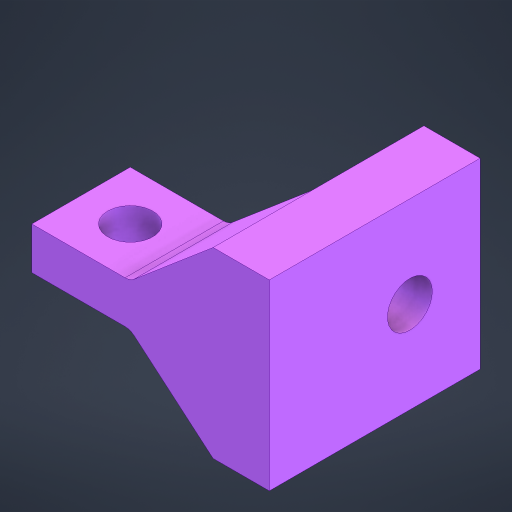
# Autodesk Inventor part: base_servos
Saved by Autodesk Inventor 2023.1 (Build 271208000, 208)
## iProperties
Created: 2022-11-08
Part Number: base_servos
Material: Generic
Document SubType Name: Modeling
Designer: amtat
Density: 1 g/cm^3
Appearance: Default
Author: amtat
Autodesk Inventor part; units mm, degrees
ref_plane "YZ Plane" through (0, 0, 0) normal (1, 0, 0) x (0, 1, 0)
ref_plane "XZ Plane" through (0, 0, 0) normal (0, 1, 0) x (-1, 0, 0)
ref_plane "XY Plane" through (0, 0, 0) normal (0, 0, 1) x (1, 0, 0)
sketch "Sketch1" plane through (0, 0, 0) normal (1, 0, 0) x (0, 1, 0)
  circle A0 centre (0, 0) radius 1.6
  line L0 (0, 0) -> (0, -66.3)
  circle A1 centre (0, -66.3) radius 1.6
  line L1 (0, 0) -> (3.5, 0)
  line L2 (3.5, 0) -> (3.5, 3.5)
  line L3 (3.5, 3.5) -> (-3.5, 3.5)
  line L4 (-3.5, 3.5) -> (-3.5, -3.5)
  line L5 (-3.5, -3.5) -> (3.5, -3.5)
  line L6 (3.5, -3.5) -> (3.5, 0)
  line L7 (0, -66.3) -> (3.5, -66.3)
  line L8 (3.5, -66.3) -> (3.5, -62.8)
  line L9 (3.5, -62.8) -> (-3.5, -62.8)
  line L10 (-3.5, -62.8) -> (-3.5, -69.8)
  line L11 (-3.5, -69.8) -> (3.5, -69.8)
  line L12 (3.5, -69.8) -> (3.5, -66.3)
  line L13 (3.5, 3.5) -> (3.5, 6.5)
  line L14 (3.5, 6.5) -> (-3.5, 6.5)
  line L15 (-3.5, 6.5) -> (-3.5, 3.5)
  line L16 (3.5, -69.8) -> (3.5, -72.8)
  line L17 (3.5, -72.8) -> (-3.5, -72.8)
  line L18 (-3.5, -72.8) -> (-3.5, -69.8)
  dimension "d0" = 3.2
  dimension "d1" = 66.3
  dimension "d2" = 3.2
  dimension "d3" = 3.5
  dimension "d4" = 3.5
  dimension "d5" = 7
  dimension "d6" = 7
  dimension "d7" = 3.5
  dimension "d8" = 3.5
  dimension "d9" = 7
  dimension "d10" = 7
  dimension "d11" = 3
  dimension "d12" = 3
  constraints: 38 end point, 11 perpendicular, 8 point on line, 2 centre point, 2 coincident, 2 vertical, 1 horizontal
  measures "d0" diameter of A0
  measures "d1" distance of L0.start L0.end
  measures "d2" diameter of A1
  measures "d3" distance of L0.start L1.end
  measures "d4" distance of L1.end L2.end
  measures "d5" distance of L2.end L3.end
  measures "d6" distance of L3.end L4.end
  measures "d7" distance of L7.start L7.end
  measures "d8" distance of L7.end L8.end
  measures "d9" distance of L8.end L9.end
  measures "d10" distance of L9.end L10.end
  measures "d11" distance of L2.end L13.end
  measures "d12" distance of L11.end L16.end
extrude "Extrusion1" add sketch "Sketch1" along normal blind 3 contours L1 L6 L5 L0 A0 | A0 L0 L5 L4 L3 L2 L1 | L3 L15 L14 L13 | L9 L8 L7 A1 L0 | L0 A1 L7 L12 L11 L10 L9 | L11 L16 L17 L18
sketch "Sketch2" plane through (3, 0, 0) normal (1, 0, 0) x (0, 0, -1)
  line L0 (-6.5, 3.5) -> (-6.5, -3.5) projected
  line L1 (-6.5, -3.5) -> (3.5, -3.5) projected
  line L2 (3.5, -3.5) -> (3.5, 3.5) projected
  line L3 (3.5, 3.5) -> (-6.5, 3.5) projected
  circle A0 centre (0, 0) radius 1.6 projected
  line L4 (62.8, -3.5) -> (72.8, -3.5) projected
  line L5 (72.8, -3.5) -> (72.8, 3.5) projected
  line L6 (72.8, 3.5) -> (62.8, 3.5) projected
  line L7 (62.8, 3.5) -> (62.8, -3.5) projected
  circle A1 centre (66.3, 0) radius 1.6 projected
  line L8 (-6.5, 3.5) -> (-6.5, -3.5) projected
  line L9 (-6.5, 3.5) -> (-2.5, 3.5)
  line L10 (3.5, 3.5) -> (-6.5, 3.5) projected
  line L11 (-2.5, 3.5) -> (-2.5, -3.5)
  line L12 (-6.5, -3.5) -> (3.5, -3.5) projected
  line L13 (-2.5, -3.5) -> (-6.5, -3.5)
  line L14 (72.8, 3.5) -> (68.8, 3.5)
  line L15 (72.8, 3.5) -> (62.8, 3.5) projected
  line L16 (68.8, 3.5) -> (68.8, -3.5)
  line L17 (62.8, -3.5) -> (72.8, -3.5) projected
  line L18 (72.8, -3.5) -> (68.8, -3.5)
  dimension "d15" = 4
  dimension "d16" = 4
  constraints: 12 end point, 4 point on line, 2 collinear, 2 perpendicular
  measures "d15" distance of L0.start L9.end
  measures "d16" distance of L5.end L14.end
extrude "Extrusion2" add sketch "Sketch2" along normal blind 10 contours L3 L11 L1 L0 | L16 L6 L5 L4
sketch "Sketch3" plane through (0, 0, 0) normal (-1, 0, 0) x (0, 0, 1)
  line L0 (6.5, 3.5) -> (6.5, -3.5) projected
  line L1 (-3.5, 3.5) -> (6.5, 3.5) projected
  line L2 (-3.5, -3.5) -> (-3.5, 3.5) projected
  line L3 (6.5, -3.5) -> (-3.5, -3.5) projected
  circle A0 centre (0, 0) radius 1.6 projected
extrude "Extrusion3" cut sketch "Sketch3" against normal through all
sketch "Sketch4" plane through (0, -3.5, -72.8) normal (0, -1, 0) x (1, 0, 0)
  line L0 (0, 10) -> (0, 0) projected
  line L1 (0, 0) -> (13, 0) projected
  line L2 (13, 4) -> (13, 0) projected
  line L3 (3, 4) -> (13, 4) projected
  line L4 (3, 10) -> (3, 4) projected
  line L5 (0, 10) -> (3, 10) projected
  point P0 (0, 72.8)
extrude "Extrusion4" add sketch "Sketch4" along normal blind 3
sketch "Sketch5" plane through (0, 3.5, -62.8) normal (0, 1, 0) x (1, 0, 0)
  line L0 (0, 10) -> (0, 0) projected
  line L1 (0, 0) -> (3, 0) projected
  line L2 (3, 6) -> (3, 0) projected
  line L3 (3, 6) -> (13, 6) projected
  line L4 (13, 10) -> (13, 6) projected
  line L5 (0, 10) -> (13, 10) projected
  point P0 (0, -62.8)
extrude "Extrusion5" add sketch "Sketch5" along normal blind 3
sketch "Sketch6" plane through (13, 0, 0) normal (1, 0, 0) x (0, 0, -1)
  line L0 (68.8, -6.5) -> (68.8, 6.5) projected
  line L1 (72.8, -6.5) -> (68.8, -6.5) projected
  line L2 (72.8, 6.5) -> (72.8, -6.5) projected
  line L3 (68.8, 6.5) -> (72.8, 6.5) projected
  point P0 (0, 0)
extrude "Extrusion6" cut sketch "Sketch6" against normal blind 2
sketch "Sketch7" plane through (0, -6.5, -72.8) normal (0, 0, -1) x (-1, 0, 0)
  line L0 (0, 0) -> (-11, 0) projected
  line L1 (-11, 0) -> (-7, 0)
  line L2 (-7, 0) -> (-7, 13.1195)
  line L3 (-3, 0) -> (-3, 13) projected
  line L4 (-11, 13) -> (-11, 0) projected
  line L5 (0, 0) -> (-11, 0) projected
  line L6 (0, 13) -> (0, 0) projected
  line L7 (-11, 13) -> (0, 13) projected
  point P0 (0, 6.5)
  point P1 (-7, 13)
  dimension "d27" = 4
  constraints: 4 end point, 1 perpendicular, 1 point on line
  measures "d27" distance of L0.end L1.end
extrude "Extrusion7" add sketch "Sketch7" along normal blind 6 contours L0 L4 L7 L2
sketch "Sketch8" plane through (7, -6.5, -72.8) normal (-1, 0, 0) x (0, 0, 1)
  line L0 (0, 13) -> (0, 0) projected
  line L1 (0, 13) -> (-6, 13) projected
  line L2 (-6, 0) -> (-6, 13) projected
  line L3 (0, 0) -> (-6, 0) projected
  line L4 (-6, 13) -> (-6, 0) projected
  line L5 (-6, 0) -> (-6, 6.5)
  line L6 (-6, 6.5) -> (-3, 6.5)
  circle A0 centre (-3, 6.5) radius 1.6
  point P0 (72.8, 6.5)
  dimension "d30" = 6.5
  dimension "d31" = 3
  dimension "d32" = 3.2
  constraints: 4 end point, 1 centre point, 1 coincident, 1 midpoint, 1 perpendicular
  measures "d30" distance of L2.start L5.end
  measures "d31" distance of L5.end L6.end
  measures "d32" diameter of A0
extrude "Extrusion8" cut sketch "Sketch8" against normal blind 6 contours A0
sketch "Sketch9" plane through (3, 0, 0) normal (1, 0, 0) x (0, 0, -1)
  circle A0 centre (66.3, 0) radius 1.6 projected
  line L0 (68.8, -6.5) -> (68.8, 6.5) projected
  line L1 (62.8, 6.5) -> (68.8, 6.5) projected
  line L2 (62.8, -6.5) -> (62.8, 6.5) projected
  line L3 (68.8, -6.5) -> (62.8, -6.5) projected
  point P0 (0, 0)
extrude "Extrusion9" cut sketch "Sketch9" against normal blind 6
sketch "Sketch10" plane through (0, 0, 0) normal (-1, 0, 0) x (0, 0, 1)
  line L0 (-68.8, -6.5) -> (-68.8, 6.5) projected
  line L1 (-72.8, 6.5) -> (-68.8, 6.5) projected
  line L2 (-72.8, 6.5) -> (-72.8, -6.5) projected
  line L3 (-68.8, -6.5) -> (-72.8, -6.5) projected
  point P0 (0, 0)
extrude "Extrusion10" add sketch "Sketch10" along normal blind 5.9
sketch "Sketch11" plane through (7, -6.5, -72.8) normal (0, 0, -1) x (-1, 0, 0)
  line L0 (0, 13) -> (0, 0) projected
  line L1 (0, 0) -> (12.9, 0) projected
  line L2 (12.9, 13) -> (12.9, 0) projected
  line L3 (0, 13) -> (12.9, 13) projected
  line L4 (-4, 0) -> (12.9, 0) projected
  line L5 (12.9, 0) -> (12.9, 5)
  line L6 (12.9, 13) -> (12.9, 0) projected
  line L7 (12.9, 5) -> (12.9, 8)
  line L8 (12.9, 8) -> (6.9, 8)
  line L9 (0, 0) -> (0, 13) projected
  line L10 (6.9, 8) -> (0, 13)
  line L11 (12.9, 5) -> (6.9, 5)
  line L12 (-4, 0) -> (0, 0) projected
  line L13 (6.9, 5) -> (0, 0)
  point P0 (7, 6.5)
  dimension "d39" = 5
  dimension "d40" = 3
  dimension "d41" = 6
  constraints: 12 end point, 2 point on line, 1 horizontal, 1 perpendicular
  measures "d39" distance of L1.end L5.end
  measures "d40" distance of L5.end L7.end
  measures "d41" distance of L7.end L8.end
extrude "Extrusion11" cut sketch "Sketch11" against normal blind 5.9 contours L3 L2 L8 L10 | L13 L11 L2 L1
sketch "Sketch12" plane through (11, -6.5, -68.8) normal (0, 0, 1) x (1, 0, 0)
  line L0 (-10.9, 5) -> (-4, 0) projected
  line L1 (0, 0) -> (-4, 0) projected
  line L2 (0, 0) -> (0, 13) projected
  line L3 (0, 13) -> (-4, 13) projected
  line L4 (-4, 13) -> (-10.9, 8) projected
  line L5 (-10.9, 8) -> (-16.9, 8) projected
  line L6 (-16.9, 5) -> (-16.9, 8) projected
  line L7 (-16.9, 5) -> (-10.9, 5) projected
  point P0 (-11, 6.5)
extrude "Extrusion12" add sketch "Sketch12" along normal blind 3
sketch "Sketch13" plane through (-5.9, -1.5, -72.8) normal (0, -1, 0) x (1, 0, 0)
  line L0 (6, 0) -> (0, 0) projected
  line L1 (0, 0) -> (0, 3.5)
  line L2 (0, 0) -> (0, 7) projected
  line L3 (0, 0) -> (0, 7) projected
  line L4 (6, 0) -> (0, 0) projected
  line L5 (6, 0) -> (6, 7) projected
  line L6 (0, 7) -> (6, 7) projected
  line L7 (0, 3.5) -> (3.5, 3.5)
  circle A0 centre (3.5, 3.5) radius 1.6
  point P0 (5.9, 72.8)
  dimension "d46" = 3.5
  dimension "d47" = 3.5
  dimension "d48" = 3.2
  constraints: 4 end point, 1 centre point, 1 coincident, 1 horizontal, 1 midpoint
  measures "d46" distance of L0.end L1.end
  measures "d47" distance of L1.end L7.end
  measures "d48" diameter of A0
extrude "Extrusion13" cut sketch "Sketch13" against normal through all contours A0
sketch "Sketch14" plane through (11, -6.5, -65.8) normal (0, 0, 1) x (1, 0, 0)
  line L0 (-10.9, 5) -> (-4, 0) projected
  line L1 (-4, 0) -> (0, 0) projected
  line L2 (0, 0) -> (0, 13) projected
  line L3 (0, 13) -> (-4, 13) projected
  line L4 (-4, 13) -> (-10.9, 8) projected
  line L5 (-10.9, 8) -> (-16.9, 8) projected
  line L6 (-16.9, 8) -> (-16.9, 5) projected
  line L7 (-16.9, 5) -> (-10.9, 5) projected
  line L8 (-4, 13) -> (-10.9, 8) projected
  line L9 (-10.9, 8) -> (-9.9, 8)
  line L10 (-9.9, 8) -> (-4, 13)
  line L11 (-4, 0) -> (-10.9, 5) projected
  line L12 (-10.9, 5) -> (-9.9, 5)
  line L13 (-9.9, 5) -> (-4, 0)
  point P0 (-11, 6.5)
  dimension "d52" = 1
  constraints: 8 end point, 2 horizontal
  measures "d52" distance of L4.end L9.end
extrude "Extrusion14" cut sketch "Sketch14" against normal blind 10 contours L12 L13 L0 | L4 L10 L9
sketch "Sketch15" plane through (0, -6.5, -78.8) normal (0, 0, -1) x (-1, 0, 0)
  line L0 (-11, 0) -> (-7, 0) projected
  line L1 (-7, 0) -> (-7, 13) projected
  line L2 (-7, 13) -> (-11, 13) projected
  line L3 (-11, 13) -> (-11, 0) projected
  point P0 (0, 6.5)
extrude "Extrusion15" add sketch "Sketch15" along normal blind 2
fillet "Fillet2" radius 1 2 edges at (1.1, 1.5, -69.3) (1.1, -1.5, -69.3)
body "Solid1"
